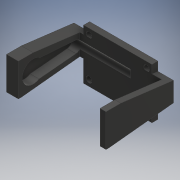
# Autodesk Inventor part: soporteCamaraB
Saved by Autodesk Inventor 2017 (Build 210142000, 142)
## iProperties
Part Number: soporteCamaraB
Material: Genérico
Document SubType Name: Modeling
Designer: Roberto
Density: 1 g/cm^3
Appearance: Valor por defecto
Author: Roberto
Autodesk Inventor part; units mm, degrees
ref_plane "YZ Plane" through (0, 0, 0) normal (1, 0, 0) x (0, 1, 0)
ref_plane "XZ Plane" through (0, 0, 0) normal (0, 1, 0) x (-1, 0, 0)
ref_plane "XY Plane" through (0, 0, 0) normal (0, 0, 1) x (1, 0, 0)
sketch "Boceto1" plane through (0, 0, 0) normal (1, 0, 0) x (0, 1, 0)
  arc A0 (0.2295, 0.2896) -> (0.1967, -0.3128) centre (0, 0) ccw
  arc A1 (1.4408, -0.1992) -> (1.4375, 0.1994) centre (1.4226, 0) ccw
  line L0 (0.2295, 0.2896) -> (1.4375, 0.1994)
  line L1 (0.1967, -0.3128) -> (1.4408, -0.1992)
  circle A2 centre (0, 0) radius 0.3
  line L2 (0, 0) -> (0, 0.55)
  line L3 (1.7726, 0.3309) -> (0, 0.55)
  line L4 (0, 0.55) -> (-0.5, 0.55)
  line L5 (-0.5, 0.55) -> (-0.5, 0)
  line L6 (1.7726, -0.3258) -> (-0.4, -0.55)
  line L7 (-0.4, -0.55) -> (-0.5, -0.55)
  line L8 (-0.5, -0.55) -> (-0.5, 0)
  line L9 (1.6226, 0.0017) -> (1.7726, 0.0017)
  line L10 (1.7726, 0.0017) -> (1.7726, 0.3309)
  line L11 (1.7726, 0.3309) -> (1.7726, -0.3258)
  dimension "d0" = 0.55
  dimension "d3" = 0.5
  constraints: 24 end point, 5 point on circle, 3 centre point, 2 perpendicular, 1 horizontal, 1 vertical
  measures "d0" distance of L2.start L2.end
  measures "d3" distance of L2.end L4.end
extrude "Extrusión1" add sketch "Boceto1" along normal blind 0.4 contours A0 L2 L3 L10 L9 A1 L0 | A0 L1 A1 L9 L11 L6 L7 L8 L5 L4 L2
sketch "Boceto2" plane through (0, 0, 0) normal (-1, 0, 0) x (0, 0, 1)
  line L0 (0.1994, 1.4375) -> (0.2896, 0.2295) projected
  arc A0 (-0.3128, 0.1967) -> (0.2896, 0.2295) centre (0, 0) ccw projected
  line L1 (-0.3128, 0.1967) -> (-0.1992, 1.4408) projected
  arc A1 (0.1994, 1.4375) -> (-0.1992, 1.4408) centre (0, 1.4226) ccw projected
  line L2 (0.3309, 1.7726) -> (0.55, 0) projected
  line L3 (-0.55, -0.4) -> (-0.3258, 1.7726) projected
  line L4 (-0.55, -0.5) -> (-0.55, -0.4) projected
  line L5 (0.55, -0.5) -> (-0.55, -0.5) projected
  line L6 (0.55, 0) -> (0.55, -0.5) projected
  line L7 (-0.3258, 1.7726) -> (0.3309, 1.7726) projected
extrude "Extrusión2" add sketch "Boceto2" against normal blind 0.1 contours L0 A0 L1 A1
sketch "Boceto3" plane through (0.4, 0, 0) normal (1, 0, 0) x (0, 0, -1)
  line L0 (-0.3, 2.0226) -> (0.3, 2.0226) projected
  line L1 (-0.3309, 1.7726) -> (-0.55, 0) projected
  line L2 (0.55, -0.4) -> (0.3258, 1.7726) projected
  line L3 (-0.3309, 1.7726) -> (-0.55, 0) projected
  line L4 (-0.3309, 1.7726) -> (0.3258, 1.7726)
  line L5 (0.55, -0.4) -> (0.3258, 1.7726) projected
  line L6 (0.2897, 1.5726) -> (0.2691, 1.7726)
  line L7 (0.3464, 1.5726) -> (-0.3556, 1.5726)
  line L8 (-0.3309, 1.7726) -> (-0.3556, 1.5726)
  line L9 (0.3258, 1.7726) -> (0.3464, 1.5726)
  point P0 (0, 0)
  point P1 (-0.3068, 1.9676)
  constraints: 10 end point, 5 point on line, 2 horizontal, 1 parallel
extrude "Extrusión3" add sketch "Boceto3" along normal blind 2.75
sketch "Boceto4" plane through (3.15, 0, 0) normal (1, 0, 0) x (0, 0, -1)
  line L0 (-0.3556, 1.5726) -> (-0.55, 0) projected
  line L1 (-0.55, 0) -> (-0.55, -0.5) projected
  line L2 (-0.55, -0.5) -> (0.55, -0.5) projected
  line L3 (0.55, -0.5) -> (0.55, -0.4) projected
  line L4 (0.55, -0.4) -> (0.3464, 1.5726) projected
  line L5 (-0.2896, 0.2295) -> (-0.1994, 1.4375) projected
  arc A0 (-0.1323, 1.5726) -> (-0.1994, 1.4375) centre (0, 1.4226) ccw projected
  line L6 (0.1992, 1.4408) -> (0.3128, 0.1967) projected
  arc A1 (-0.2896, 0.2295) -> (0.3128, 0.1967) centre (0, 0) ccw projected
  line L7 (0.3258, 1.7726) -> (-0.3309, 1.7726) projected
  line L8 (-0.3556, 1.5726) -> (0.3464, 1.5726) projected
  line L9 (-0.3309, 1.7726) -> (-0.3556, 1.5726) projected
  line L10 (0.3464, 1.5726) -> (0.1323, 1.5726) projected
  arc A2 (0.1992, 1.4408) -> (0.1323, 1.5726) centre (0, 1.4226) ccw projected
  line L11 (-0.1323, 1.5726) -> (-0.3556, 1.5726) projected
  line L12 (0.3464, 1.5726) -> (0.3258, 1.7726) projected
  line L13 (-0.3309, 1.7726) -> (-0.55, 0) projected
  line L14 (0.3258, 1.7726) -> (-0.3309, 1.7726) projected
  line L15 (0.55, -0.4) -> (0.3258, 1.7726) projected
  line L16 (0.55, -0.5) -> (0.55, -0.4) projected
  line L17 (-0.55, -0.5) -> (0.55, -0.5) projected
  line L18 (-0.55, 0) -> (-0.55, -0.5) projected
  line L19 (0.3464, 1.5726) -> (0.1323, 1.5726) projected
  arc A3 (0.1992, 1.4408) -> (0.1323, 1.5726) centre (0, 1.4226) ccw projected
  line L20 (0.1992, 1.4408) -> (0.3128, 0.1967) projected
  arc A4 (-0.2896, 0.2295) -> (0.3128, 0.1967) centre (0, 0) ccw projected
  line L21 (-0.2896, 0.2295) -> (-0.1994, 1.4375) projected
  arc A5 (-0.1323, 1.5726) -> (-0.1994, 1.4375) centre (0, 1.4226) ccw projected
  line L22 (-0.1323, 1.5726) -> (-0.3556, 1.5726) projected
  line L23 (-0.3556, 1.5726) -> (-0.55, 0) projected
  line L24 (-0.55, 0) -> (-0.55, -0.5) projected
  line L25 (-0.55, -0.5) -> (0.55, -0.5) projected
  line L26 (0.55, -0.5) -> (0.55, -0.4) projected
  line L27 (0.55, -0.4) -> (0.3464, 1.5726) projected
extrude "Extrusión4" add sketch "Boceto4" along normal blind 0.2
sketch "Boceto5" plane through (3.15, 0, 0) normal (-1, 0, 0) x (0, 0, 1)
  line L0 (0.2896, 0.2295) -> (0.1994, 1.4375) projected
  arc A0 (-0.3128, 0.1967) -> (0.2896, 0.2295) centre (0, 0) ccw projected
  line L1 (-0.1992, 1.4408) -> (-0.3128, 0.1967) projected
  arc A1 (0.1994, 1.4375) -> (-0.1992, 1.4408) centre (0, 1.4226) ccw projected
  circle A2 centre (0, 0) radius 0.3695
  circle A3 centre (0, 0) radius 0.15
  dimension "d13" = 0.3
  constraints: 2 centre point, 2 coincident, 1 concentric
  measures "d13" diameter of A3
extrude "Extrusión5" add sketch "Boceto5" along normal blind 0.07 contours A3
chamfer "Chaflán1" distance 0.07 angle 45 1 edges at (3.08, 0, -0.15)
sketch "Boceto8" plane through (0, 1.7726, 0.3309) normal (0, 1, 0) x (1, 0, 0)
  line L0 (3.35, 0.6567) -> (3.35, 0) projected
  circle A0 centre (0.705, 1.2) radius 0.1
  circle A1 centre (2.645, 1.2) radius 0.1
  line L1 (2.825, -0.3) -> (2.825, 1.4)
  line L2 (0.525, 1.4) -> (0.525, -0.3)
  line L3 (0.525, -0.3) -> (0.525, 1.2)
  line L4 (0.525, -0.1) -> (0.705, -0.1)
  circle A2 centre (0.705, -0.1) radius 0.1
  circle A3 centre (2.645, -0.1) radius 0.1
  line L5 (0.525, -0.3) -> (0.525, -0.1)
  line L6 (0.525, -0.3) -> (2.825, -0.3)
  line L7 (2.645, -0.1) -> (2.645, 0)
  line L8 (2.645, 0) -> (0.705, 0)
  line L9 (0, 0) -> (3.35, 0) projected
  line L10 (3.35, 0) -> (0, 0)
  line L11 (2.645, -0.1) -> (2.645, 1.2)
  line L12 (0.525, 1.4) -> (2.825, 1.4)
  dimension "d65" = 0.2
  dimension "d63" = 0.2
  dimension "d64" = 0.18
  dimension "d66" = 1.5
  dimension "d67" = 0.2
  constraints: 22 end point, 2 centre point, 2 point on line, 2 vertical alignment, 1 coincident, 1 collinear, 1 horizontal, 1 parallel, 1 perpendicular, 1 vertical, 4 other
  measures "d63" distance of L6.start L4.start
  measures "d64" distance of L4.start L4.end
  measures "d66" distance of L6.start L3.end
  measures "d67" diameter of A0
extrude "Extrusión8" add sketch "Boceto8" against normal blind 0.2 contours L6 L2 L4 A2 L8 L9 L1 | L9 L8 L2 L12 L1 | L2 L9 A2 L4
sketch "Boceto9" plane through (0.1, 0, 0) normal (1, 0, 0) x (0, 0, -1)
  line L0 (-0.2896, 0.2295) -> (-0.1994, 1.4375) projected
  arc A0 (-0.2896, 0.2295) -> (0.3128, 0.1967) centre (0, 0) ccw projected
  line L1 (0.1992, 1.4408) -> (0.3128, 0.1967) projected
  arc A1 (0.1992, 1.4408) -> (-0.1994, 1.4375) centre (0, 1.4226) ccw projected
extrude "Extrusión9" cut sketch "Boceto9" along normal blind 2
